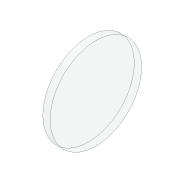
# Autodesk Inventor part: Lens
Saved by Autodesk Inventor 2020.3 (Build 243373000, 373)
## iProperties
Created: 2021-09-09
Part Number: Lens
Material: Glass
Document SubType Name: Modeling
Designer: Yusuf
Mass: 22.3312 g
Surface Area: 45.7381 cm^2
Volume: 10.2437 cm^3
Density: 2.18 g/cm^3
Appearance: Clear
Author: Yusuf
Autodesk Inventor part; units mm, degrees
ref_plane "YZ Plane" through (0, 0, 0) normal (1, 0, 0) x (0, 1, 0)
ref_plane "XZ Plane" through (0, 0, 0) normal (0, 1, 0) x (-1, 0, 0)
ref_plane "XY Plane" through (0, 0, 0) normal (0, 0, 1) x (1, 0, 0)
sketch "Sketch1" plane through (0, 0, 0) normal (0, 1, 0) x (-1, 0, 0)
  line L0 (0, 0) -> (0, 25)
  line L1 (0, 25) -> (4, 25)
  arc A0 (4, -25) -> (4, 25) centre (-123.5735, 0) ccw
  line L2 (6.4265, 0) -> (0, 0)
  dimension "d0" = 25
  dimension "d1" = 4
  dimension "d2" = 50
  dimension "d3" = 130
  constraints: 6 end point, 3 point on circle, 1 centre point, 1 horizontal, 1 perpendicular, 1 vertical
  measures "d0" distance of L0.start L0.end
  measures "d1" distance of L0.end L1.end
  measures "d2" distance of L1.end A0.start
  measures "d3" radius of A0
revolve "Revolution1" add sketch "Sketch1" angle 360 about axis through (-6.4265, 0, 0) along (1, 0, 0)
body "Solid1"
